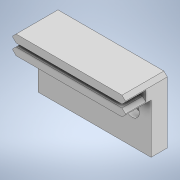
# Autodesk Inventor part: Floor_support_dammy
Saved by Autodesk Inventor 2020.4 (Build 244396010, 396A)
## iProperties
Created: 2019-05-27
Part Number: Floor_support_dammy
Material: Generic
Document SubType Name: Modeling
Designer: Dammy
Density: 1 g/cm^3
Appearance: Default
Author: Dammy
Autodesk Inventor part; units mm, degrees
ref_plane "YZ Plane" through (0, 0, 0) normal (1, 0, 0) x (0, 1, 0)
ref_plane "XZ Plane" through (0, 0, 0) normal (0, 1, 0) x (-1, 0, 0)
ref_plane "XY Plane" through (0, 0, 0) normal (0, 0, 1) x (1, 0, 0)
sketch "Sketch1" plane through (0, 0, 0) normal (0, 0, 1) x (1, 0, 0)
  line L0 (33, -19) -> (-33, -19)
  line L1 (-33, -19) -> (-33, 19)
  line L2 (-33, 19) -> (33, 19)
  line L3 (33, 19) -> (33, -19)
  line L4 (33, -19) -> (-33, 19) construction
  line L5 (-33, -19) -> (33, 19) construction
  point P0 (0, 0)
  dimension "d0" = 66
  dimension "d1" = 38
  constraints: 12 end point, 2 midpoint, 2 parallel, 1 horizontal, 1 perpendicular
  measures "d0" distance of L1.end L2.end
  measures "d1" distance of L0.end L1.end
extrude "Extrusion1" add sketch "Sketch1" along normal blind 9.5
sketch "Sketch2" plane through (0, 0, 0) normal (0, 0, -1) x (-1, 0, 0)
  line L0 (-31, -7) -> (31, -7)
  line L1 (31, -7) -> (31, -17)
  line L2 (31, -17) -> (-31, -17)
  line L3 (-31, -17) -> (-31, -7)
  line L4 (33, 19) -> (33, -19) projected
  line L5 (-33, -19) -> (-33, 19) construction
  line L6 (33, 19) -> (33, -19) construction
  line L7 (33, -19) -> (-33, -19) construction
  point P0 (0, 0)
  point P1 (0, -7)
  dimension "d4" = 2
  dimension "d5" = 2
  dimension "d6" = 12
  constraints: 8 end point, 2 parallel, 1 horizontal, 1 midpoint, 1 perpendicular, 1 vertical alignment
  measures "d4" distance between parallel lines of L4 L1
  measures "d5" distance between parallel lines of L7 L2
  measures "d6" distance between parallel lines of L7 L0
extrude "Extrusion2" cut sketch "Sketch2" against normal blind 7
sketch "Sketch3" plane through (0, 0, 9.5) normal (0, 0, 1) x (1, 0, 0)
  line L0 (33, -19) -> (33, 19) projected
  line L1 (-33, 19) -> (33, 19) construction
  line L2 (33, 19) -> (33, 8) construction
  line L3 (33, 8) -> (-33, 8) construction
  line L4 (-33, 8) -> (-33, 19) construction
  line L5 (-33, -19) -> (33, -19) projected
  line L6 (-33, 8) -> (33, 8)
  line L7 (33, 8) -> (33, 12.5)
  line L8 (33, 12.5) -> (-33, 12.5)
  line L9 (-33, 12.5) -> (-33, 8)
  line L10 (33, 19) -> (-33, 19) projected
  line L11 (-33, 19) -> (33, 19)
  line L12 (33, 19) -> (33, 14.5)
  line L13 (33, 14.5) -> (-33, 14.5)
  line L14 (-33, 14.5) -> (-33, 19)
  point P0 (0, 0)
  dimension "d9" = 27
  dimension "d10" = 2
  dimension "d11" = 4.5
  constraints: 24 end point, 6 parallel, 3 horizontal, 3 perpendicular, 3 point on line
  measures "d9" distance between parallel lines of L5 L3
  measures "d10" distance between parallel lines of L8 L13
  measures "d11" distance between parallel lines of L1 L13
extrude "Extrusion3" add sketch "Sketch3" along normal blind 15
sketch "Sketch4" plane through (0, 0, 9.5) normal (0, 0, 1) x (1, 0, 0)
  line L0 (-33, 14.5) -> (-33, 12.5) projected
  line L1 (-33, 12.5) -> (33, 12.5) projected
  line L2 (-33, 14.5) -> (33, 14.5)
  line L3 (33, 14.5) -> (33, 12.5)
  line L4 (33, 12.5) -> (-33, 12.5)
  line L5 (-33, 12.5) -> (-33, 14.5)
  point P0 (0, 0)
  constraints: 8 end point, 2 parallel, 1 horizontal, 1 perpendicular
extrude "Extrusion4" add sketch "Sketch4" along normal blind 3
chamfer "Chamfer1" distance 2 angle 45 8 edges at (33, 12.5, 18.5) (33, 8, 17) (-33, 12.5, 18.5) (-33, 8, 17) (-33, 19, 12.25) (-33, 14.5, 18.5) (33, 14.5, 18.5) (33, 19, 12.25)
sketch "Sketch5" plane through (0, 0, 9.5) normal (0, 0, 1) x (1, 0, 0)
  circle A0 centre (-22.1, 0.05) radius 5.5
  circle A1 centre (21.9, 0.05) radius 5.5
  line L0 (33, -19) -> (33, 10) projected
  line L1 (-33, -19) -> (33, -19) projected
  point P0 (0, 0)
  dimension "d19" = 11
  dimension "d20" = 11
  dimension "d21" = 44
  dimension "d22" = 11.1
  dimension "d23" = 19.05
  constraints: 2 centre point, 1 horizontal alignment
  measures "d19" diameter of A0
  measures "d20" diameter of A1
  measures "d21" distance of A1.centre A0.centre
  measures "d22" distance from line of L0 A1.centre
  measures "d23" distance from line of L1 A1.centre
hole "Hole1" at (-22.1, 0.05, 9.5) at (21.9, 0.05, 9.5) direction (0, 0, -1) diameter 5.5 end through all counterbore diameter 8.5 counterbore depth 5
equation "\"d11\" = -0.5 * d10 + 0.5 * d1 - 0.5 * d9"
equation "\"d20\" = d19"
body "Solid1"
